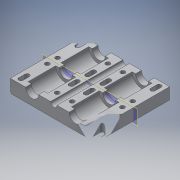
# Autodesk Inventor part: AXCARv4
Saved by Autodesk Inventor 2016 (Build 200138000, 138)
## iProperties
Created: 2015-07-22
Part Number: AXCARv4
Material: PC/ABS Plastic
Document SubType Name: Modeling
Designer: Jose
Density: 0.357273 g/cm^3
Appearance: Smooth - White
Mass: 84.7102 g
Surface Area: 389.676 cm^2
Volume: 154.019 cm^3
Author: Jose
Autodesk Inventor part; units mm, degrees
ref_plane "YZ Plane" through (0, 0, 0) normal (1, 0, 0) x (0, 1, 0)
ref_plane "XZ Plane" through (0, 0, 0) normal (0, 1, 0) x (-1, 0, 0)
ref_plane "XY Plane" through (0, 0, 0) normal (0, 0, 1) x (1, 0, 0)
sketch "Sketch1" plane through (0, 0, 0) normal (0, 0, 1) x (1, 0, 0)
  line L0 (-60, 50) -> (60, 50)
  line L1 (60, 50) -> (60, -50)
  line L2 (60, -50) -> (-60, -50)
  line L3 (-60, -50) -> (-60, 50)
  point P0 (0, 0)
  point P1 (-60, 0)
  point P2 (0, 50)
  dimension "d0" = 120
  dimension "d1" = 100
  constraints: 8 end point, 2 midpoint, 2 parallel, 1 horizontal, 1 horizontal alignment, 1 perpendicular, 1 vertical alignment
  measures "d0" distance of L0.start L0.end
  measures "d1" distance of L0.end L1.end
extrude "Extrusion1" add sketch "Sketch1" along normal blind 18
sketch "Sketch2" plane through (-60, 50, 0) normal (0, 1, 0) x (1, 0, 0)
  line L0 (0, 0) -> (120, 0) projected
  line L1 (0, 0) -> (0, -18) projected
  line L2 (120, -18) -> (0, -18) projected
  line L3 (120, 0) -> (120, -18) projected
  line L4 (120, -18) -> (0, -18) projected
  circle A0 centre (30, -18) radius 13.75
  circle A1 centre (90, -18) radius 13.75
  circle A2 centre (60, -18) radius 4.5
  point P0 (60, 0)
  dimension "d4" = 27.5
  dimension "d5" = 9
  dimension "d11" = 30
  dimension "d12" = 30
  constraints: 3 centre point, 2 point on line, 1 equal radius, 1 midpoint
  measures "d4" diameter of A0
  measures "d5" diameter of A2
  measures "d11" distance of A2.centre A1.centre
  measures "d12" distance of A2.centre A0.centre
extrude "Extrusion2" cut sketch "Sketch2" against normal through all contours A0 L2 | L2 A0 | A1 L2 | L2 A1 | A2 L2 | L2 A2
sketch "Sketch3" plane through (0, 0, 18) normal (0, 0, 1) x (1, 0, 0)
  line L0 (16.25, -50) -> (16.25, 50) projected
  line L1 (16.25, 50) -> (4.5, 50) projected
  line L2 (4.5, 50) -> (4.5, -50) projected
  line L3 (4.5, -50) -> (16.25, -50) projected
  line L4 (-4.5, -50) -> (-4.5, 50) projected
  line L5 (-4.5, 50) -> (-16.25, 50) projected
  line L6 (-16.25, 50) -> (-16.25, -50) projected
  line L7 (-16.25, -50) -> (-4.5, -50) projected
  line L8 (-43.75, -50) -> (-43.75, 50) projected
  line L9 (-43.75, 50) -> (-60, 50) projected
  line L10 (-60, 50) -> (-60, -50) projected
  line L11 (-60, -50) -> (-43.75, -50) projected
  line L12 (43.75, 50) -> (43.75, -50) projected
  line L13 (43.75, -50) -> (60, -50) projected
  line L14 (60, -50) -> (60, 50) projected
  line L15 (60, 50) -> (43.75, 50) projected
  line L16 (-60, 50) -> (60, 50) construction
  line L17 (-51.875, 50) -> (-51.875, -50) construction
  line L18 (51.875, 50) -> (51.875, -50) construction
  line L19 (16.25, 50) -> (4.5, 50) construction
  line L20 (10.375, 50) -> (10.375, -50) construction
  line L21 (4.5, -50) -> (16.25, -50) construction
  line L22 (-10.375, 50) -> (-10.375, -50) construction
  line L23 (-16.25, -50) -> (-4.5, -50) construction
  circle A0 centre (-51.875, 35) radius 3.05
  circle A1 centre (-51.875, -35) radius 3.05
  circle A2 centre (51.875, 35) radius 3.05
  circle A3 centre (51.875, -35) radius 3.05
  circle A4 centre (-10.375, 35) radius 3.05
  circle A5 centre (10.375, 35) radius 3.05
  circle A6 centre (-10.375, -35) radius 3.05
  circle A7 centre (10.375, -35) radius 3.05
  dimension "d13" = 15
  dimension "d14" = 15
  dimension "d15" = 6.1
  constraints: 8 centre point, 8 end point, 8 point on line, 7 equal radius, 6 horizontal alignment, 5 midpoint, 4 other
  measures "d13" distance of L17.start A0.centre
  measures "d14" distance of L17.end A1.centre
  measures "d15" diameter of A4
extrude "Extrusion3" cut sketch "Sketch3" against normal through all contours A0 | A1 | A2 | A3 | A4 | A5 | A6 | A7
sketch "Sketch6" plane through (0, 0, 0) normal (0, 0, -1) x (-1, 0, 0)
  circle A0 centre (-51.875, 35) radius 3.05 projected
  circle A1 centre (51.875, 35) radius 3.05 projected
  circle A2 centre (10.375, 35) radius 3.05 projected
  circle A3 centre (-10.375, 35) radius 3.05 projected
  circle A4 centre (-10.375, -35) radius 3.05 projected
  circle A5 centre (10.375, -35) radius 3.05 projected
  circle A6 centre (51.875, -35) radius 3.05 projected
  circle A7 centre (-51.875, -35) radius 3.05 projected
  line L0 (60, 50) -> (-60, 50) projected
  line L1 (-60, 50) -> (-60, -50) projected
  line L2 (-60, -50) -> (60, -50) projected
  line L3 (60, -50) -> (60, 50) projected
  line L4 (51.875, 7.125) -> (-51.875, 7.125) construction
  line L5 (-51.875, 7.125) -> (-51.875, -7.125) construction
  line L6 (-51.875, -7.125) -> (51.875, -7.125) construction
  line L7 (51.875, -7.125) -> (51.875, 7.125) construction
  circle A8 centre (-51.875, -7.125) radius 3.05
  circle A9 centre (51.875, -7.125) radius 3.05
  circle A10 centre (10.375, -7.125) radius 3.05
  circle A11 centre (-10.375, -7.125) radius 3.05
  circle A12 centre (-10.375, 7.125) radius 3.05
  circle A13 centre (10.375, 7.125) radius 3.05
  circle A14 centre (51.875, 7.125) radius 3.05
  circle A15 centre (-51.875, 7.125) radius 3.05
  point P0 (0, 0)
  point P1 (0, 7.125)
  point P2 (51.875, 0)
  dimension "d26" = 14.25
  dimension "d27" = 6.1
  constraints: 8 centre point, 8 end point, 7 equal radius, 6 vertical alignment, 4 coincident, 4 point on line, 2 midpoint, 2 parallel, 1 horizontal, 1 horizontal alignment, 1 perpendicular
  measures "d26" distance of L6.end L4.start
  measures "d27" diameter of A14
extrude "Extrusion6" cut sketch "Sketch6" against normal through all contours A8 | A9 | A10 | A11 | A12 | A13 | A14 | A15
sketch "Sketch7" plane through (0, 0, 0) normal (0, 0, -1) x (-1, 0, 0)
  circle A0 centre (51.875, 7.125) radius 3.05 projected
  circle A1 centre (-10.375, 7.125) radius 3.05 projected
  circle A2 centre (10.375, -7.125) radius 3.05 projected
  circle A3 centre (-51.875, -7.125) radius 3.05 projected
  circle A4 centre (51.875, -7.125) radius 3.05 projected
  circle A5 centre (-10.375, -7.125) radius 3.05 projected
  circle A6 centre (10.375, 7.125) radius 3.05 projected
  circle A7 centre (-51.875, 7.125) radius 3.05 projected
  circle A8 centre (-51.875, 35) radius 3.05 projected
  circle A9 centre (51.875, 35) radius 3.05 projected
  circle A10 centre (10.375, 35) radius 3.05 projected
  circle A11 centre (-10.375, 35) radius 3.05 projected
  circle A12 centre (-10.375, -35) radius 3.05 projected
  circle A13 centre (10.375, -35) radius 3.05 projected
  circle A14 centre (51.875, -35) radius 3.05 projected
  circle A15 centre (-51.875, -35) radius 3.05 projected
  line L0 (60, 50) -> (-60, 50) projected
  line L1 (-60, 50) -> (-60, -50) projected
  line L2 (-60, -50) -> (60, -50) projected
  line L3 (60, -50) -> (60, 50) projected
  line L4 (51.875, -35) -> (51.875, -43.5) construction
  line L5 (54.925, -35) -> (54.925, -43.5)
  line L6 (48.825, -43.5) -> (48.825, -35)
  arc A16 (54.925, -35) -> (48.825, -35) centre (51.875, -35) ccw
  arc A17 (48.825, -43.5) -> (54.925, -43.5) centre (51.875, -43.5) ccw
  line L7 (-51.875, -35) -> (-51.875, -43.5) construction
  line L8 (-54.925, -35) -> (-54.925, -43.5)
  line L9 (-48.825, -43.5) -> (-48.825, -35)
  arc A18 (-48.825, -35) -> (-54.925, -35) centre (-51.875, -35) ccw
  arc A19 (-54.925, -43.5) -> (-48.825, -43.5) centre (-51.875, -43.5) ccw
  line L10 (-51.875, 35) -> (-51.875, 43.5) construction
  line L11 (-54.925, 35) -> (-54.925, 43.5)
  line L12 (-48.825, 43.5) -> (-48.825, 35)
  arc A20 (-54.925, 35) -> (-48.825, 35) centre (-51.875, 35) ccw
  arc A21 (-48.825, 43.5) -> (-54.925, 43.5) centre (-51.875, 43.5) ccw
  line L13 (51.875, 35) -> (51.875, 43.5) construction
  line L14 (54.925, 35) -> (54.925, 43.5)
  line L15 (48.825, 43.5) -> (48.825, 35)
  arc A22 (48.825, 35) -> (54.925, 35) centre (51.875, 35) ccw
  arc A23 (54.925, 43.5) -> (48.825, 43.5) centre (51.875, 43.5) ccw
  line L16 (10.375, -7.125) -> (10.375, -15.625) construction
  line L17 (13.425, -7.125) -> (13.425, -15.625)
  line L18 (7.325, -15.625) -> (7.325, -7.125)
  arc A24 (13.425, -7.125) -> (7.325, -7.125) centre (10.375, -7.125) ccw
  arc A25 (7.325, -15.625) -> (13.425, -15.625) centre (10.375, -15.625) ccw
  line L19 (-10.375, -7.125) -> (-10.375, -15.625) construction
  line L20 (-7.325, -7.125) -> (-7.325, -15.625)
  line L21 (-13.425, -15.625) -> (-13.425, -7.125)
  arc A26 (-7.325, -7.125) -> (-13.425, -7.125) centre (-10.375, -7.125) ccw
  arc A27 (-13.425, -15.625) -> (-7.325, -15.625) centre (-10.375, -15.625) ccw
  line L22 (-10.375, 7.125) -> (-10.375, 15.625) construction
  line L23 (-7.325, 7.125) -> (-7.325, 15.625)
  line L24 (-13.425, 15.625) -> (-13.425, 7.125)
  arc A28 (-13.425, 7.125) -> (-7.325, 7.125) centre (-10.375, 7.125) ccw
  arc A29 (-7.325, 15.625) -> (-13.425, 15.625) centre (-10.375, 15.625) ccw
  line L25 (10.375, 7.125) -> (10.375, 15.625) construction
  line L26 (13.425, 7.125) -> (13.425, 15.625)
  line L27 (7.325, 15.625) -> (7.325, 7.125)
  arc A30 (7.325, 7.125) -> (13.425, 7.125) centre (10.375, 7.125) ccw
  arc A31 (13.425, 15.625) -> (7.325, 15.625) centre (10.375, 15.625) ccw
  point P0 (0, 0)
  point P1 (51.875, -39.25)
  point P2 (-51.875, -39.25)
  point P3 (-51.875, 39.25)
  point P4 (51.875, 39.25)
  point P5 (10.375, -11.375)
  point P6 (-10.375, -11.375)
  point P7 (-10.375, 11.375)
  point P8 (10.375, 11.375)
  dimension "d30" = 8.5
  dimension "d31" = 3.05
  constraints: 64 end point, 32 point on circle, 32 tangent, 16 centre point, 11 parallel, 8 midpoint, 7 equal length, 7 equal radius, 4 point on line, 1 vertical
  measures "d30" distance of L7.start L7.end
  measures "d31" radius of A17
extrude "Extrusion7" cut sketch "Sketch7" against normal through all contours A1 L24 A29 L23 | L17 A25 L18 A2 | L20 A27 L21 A5 | A6 L27 A31 L26 | A8 L11 A21 L12 | A9 L15 A23 L14 | L5 A17 L6 A14 | L9 A19 L8 A15
sketch "Sketch9" plane through (-60, 50, 0) normal (0, 1, 0) x (1, 0, 0)
  arc A0 (103.75, -18) -> (76.25, -18) centre (90, -18) ccw construction
  line L0 (120, -18) -> (103.75, -18) construction
  line L1 (120, 0) -> (120, -18) construction
  line L2 (0, 0) -> (120, 0) construction
  line L3 (0, 0) -> (0, -18) construction
  line L4 (16.25, -18) -> (0, -18) construction
  arc A1 (43.75, -18) -> (16.25, -18) centre (30, -18) ccw construction
  line L5 (55.5, -18) -> (43.75, -18) construction
  arc A2 (64.5, -18) -> (55.5, -18) centre (60, -18) ccw projected
  line L6 (76.25, -18) -> (64.5, -18) construction
  circle A3 centre (90, -18) radius 8 construction
  circle A4 centre (30, -18) radius 8 construction
  arc A5 (99, -18) -> (81, -18) centre (90, -18) ccw
  arc A6 (39, -18) -> (21, -18) centre (30, -18) ccw
  line L7 (120, -18) -> (103.75, -18) projected
  line L8 (21, -18) -> (16.25, -18)
  line L9 (103.75, -18) -> (99, -18)
  line L10 (81, -18) -> (76.25, -18)
  line L11 (43.75, -18) -> (39, -18)
  arc A7 (103.75, -18) -> (76.25, -18) centre (90, -18) ccw
  arc A8 (43.75, -18) -> (16.25, -18) centre (30, -18) ccw
  point P0 (60, 0)
  dimension "d37" = 18
  constraints: 12 point on circle, 8 end point, 4 centre point, 4 coincident, 4 collinear, 3 equal radius
  measures "d37" diameter of A5
extrude "Extrusion9" add sketch "Sketch9" against normal blind 8
ref_plane "Work Plane1" through (-60, 0, 0) normal (0, 1, 0) x (1, 0, 0)
mirror "Mirror1" about plane through (-60, 0, 0) normal (0, 1, 0) of "Extrusion9"
sketch "Sketch10" plane through (-60, 0, 0) normal (0, 1, 0) x (1, 0, 0)
  line L0 (21, -18) -> (16.25, -18) projected
  arc A0 (39, -18) -> (21, -18) centre (30, -18) ccw projected
  line L1 (43.75, -18) -> (39, -18) projected
  arc A1 (43.75, -18) -> (16.25, -18) centre (30, -18) ccw projected
  line L2 (103.75, -18) -> (99, -18) projected
  arc A2 (103.75, -18) -> (76.25, -18) centre (90, -18) ccw projected
  line L3 (81, -18) -> (76.25, -18) projected
  arc A3 (99, -18) -> (81, -18) centre (90, -18) ccw projected
  point P0 (60, 0)
extrude "Extrusion10" add sketch "Sketch10" along normal mid plane 7
chamfer "Chamfer1" distance 2 angle 45 2 edges at (-60, 0, 0) (60, 0, 0)
body "Solid1"
